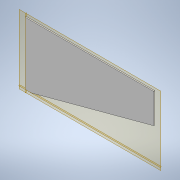
# Autodesk Inventor part: ДетальДударь
Saved by Autodesk Inventor 2020 (Build 240168000, 168)
## iProperties
Created: 2025-10-29
Part Number: ДетальДударь
Material: Типовые
Document SubType Name: Modeling
Designer: YuraD
Density: 1 g/cm^3
Appearance: По умолчанию
Author: YuraD
Autodesk Inventor part; units mm, degrees
sketch "Эскиз1" plane through (0, 0, 0) normal (0, 0, 1) x (1, 0, 0)
  line L0 (0, 613.0143) -> (0, -102.169) projected
  line L1 (-210, 0) -> (1260, 0) projected
  line L2 (0, 0) -> (50, 0)
  line L3 (1050, 510.8452) -> (0, 510.8452)
  line L4 (0, 0) -> (0, 510.8452)
  line L5 (1050, 510.8452) -> (1050, 267.9492)
  line L6 (1050, 267.9492) -> (50, 0)
  dimension "d7" = 1050
  dimension "d8" = 50
  dimension "d9" = 15
  constraints: 10 end point, 2 perpendicular, 2 point on line, 1 vertical
  measures "d7" distance between parallel lines of L5 L4
  measures "d8" distance of L2.start L2.end
  measures "d9" angle of L1 L6
extrude "Выдавливание1" add sketch "Эскиз1" along normal mid plane 10
